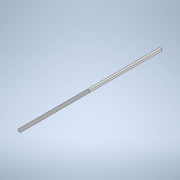
# Autodesk Inventor part: Redirection Plate
Saved by Autodesk Inventor 2020 (Build 240168000, 168)
## iProperties
Created: 2021-01-30
Part Number: Redirection Plate
Material: Generic
Document SubType Name: Modeling
Designer: magda
Density: 1 g/cm^3
Appearance: Default
Author: magda
Autodesk Inventor part; units mm, degrees
ref_plane "YZ Plane" through (0, 0, 0) normal (1, 0, 0) x (0, 1, 0)
ref_plane "XZ Plane" through (0, 0, 0) normal (0, 1, 0) x (-1, 0, 0)
ref_plane "XY Plane" through (0, 0, 0) normal (0, 0, 1) x (1, 0, 0)
sketch "Sketch1" plane through (0, 0, 0) normal (0, 0, 1) x (1, 0, 0)
  line L0 (151.8583, 166.9217) -> (156.9383, 166.9217)
  line L1 (156.9383, 166.9217) -> (156.9383, 161.8417)
  line L2 (156.9383, -10.8783) -> (-20.8617, -10.8783)
  line L3 (-20.8617, -10.8783) -> (-20.8617, 166.9217)
  line L4 (-20.8617, -5.7983) -> (151.8583, 166.9217)
  line L5 (-15.7817, -10.8783) -> (156.9383, 161.8417)
  point P0 (0, 0)
  dimension "d0" = 177.8
  dimension "d1" = 177.8
  dimension "d2" = 45
  dimension "d3" = 45
  dimension "d4" = 5.08
  dimension "d5" = 5.08
  constraints: 12 end point, 2 parallel, 2 point on line, 1 horizontal, 1 perpendicular
  measures "d0" distance of L2.start L2.end
  measures "d1" distance of L2.end L3.end
  measures "d2" angle of L5 L2
  measures "d3" angle of L4 L2
  measures "d4" distance from line of L5.start L3
  measures "d5" distance from line of L2 L4.start
extrude "Extrusion1" add sketch "Sketch1" along normal blind 177.8
body "Solid1"
